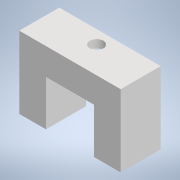
# Autodesk Inventor part: Toper_Carril
Saved by Autodesk Inventor 2022 (Build 260153000, 153)
## iProperties
Created: 2022-01-30
Part Number: Toper_Carril
Material: Generic
Document SubType Name: Modeling
Designer: katha
Density: 1 g/cm^3
Appearance: Default
Author: katha
Autodesk Inventor part; units mm, degrees
ref_plane "YZ Plane" through (0, 0, 0) normal (1, 0, 0) x (0, 1, 0)
ref_plane "XZ Plane" through (0, 0, 0) normal (0, 1, 0) x (-1, 0, 0)
ref_plane "XY Plane" through (0, 0, 0) normal (0, 0, 1) x (1, 0, 0)
sketch "Sketch1" plane through (0, 0, 0) normal (0, 0, 1) x (1, 0, 0)
  line L0 (0, 0) -> (0, 3)
  line L1 (0, 3) -> (25, 3)
  line L2 (25, 3) -> (25, 0)
  line L3 (25, 0) -> (0, 0)
  line L4 (0.5, 3.5) -> (24.5, 3.5)
  line L5 (25, 3) -> (28, 3)
  line L6 (28, 3) -> (28, -17)
  line L7 (28, -17) -> (25, -17)
  line L8 (25, -17) -> (25, 3)
  line L9 (24.5, 3.5) -> (28.5, 3.5)
  line L10 (28.5, 3.5) -> (28.5, -17.5)
  line L11 (28.5, -17.5) -> (24.5, -17.5)
  line L12 (24.5, -17.5) -> (24.5, -0.5)
  line L13 (-3, 3) -> (0, 3)
  line L14 (0, 3) -> (0, -17)
  line L15 (0, -17) -> (-3, -17)
  line L16 (-3, -17) -> (-3, 3)
  line L17 (0.5, 3.5) -> (-3.5, 3.5)
  line L18 (-3.5, 3.5) -> (-3.5, -17.5)
  line L19 (-3.5, -17.5) -> (0.5, -17.5)
  line L20 (24.5, -0.5) -> (0.5, -0.5)
  line L21 (0.5, -17.5) -> (0.5, -0.5)
  line L22 (12.5, 0) -> (12.5, -5.0944) construction
  line L23 (21.5, -3.5) -> (21.5, -20.5)
  line L24 (21.5, -20.5) -> (31.5, -20.5)
  line L25 (31.5, -20.5) -> (31.5, 6.5)
  line L26 (31.5, 6.5) -> (24.5, 6.5)
  line L27 (24.5, 6.5) -> (0.5, 6.5)
  line L28 (0.5, 6.5) -> (-6.5, 6.5)
  line L29 (-6.5, 6.5) -> (-6.5, -20.5)
  line L30 (-6.5, -20.5) -> (3.5, -20.5)
  line L31 (3.5, -20.5) -> (3.5, -3.5)
  line L32 (3.5, -3.5) -> (21.5, -3.5)
  dimension "d1" = 0.5
  dimension "d3" = 0.5
  dimension "d4" = 0.5
  dimension "d5" = 3
  constraints: 66 end point, 8 vertical, 6 horizontal, 3 equal length, 1 midpoint, 22 other
  measures "d1" distance between parallel lines of L8 L12
  measures "d3" distance between parallel lines of L7 L11
  measures "d4" distance between parallel lines of L20 L3
  measures "d5" distance between parallel lines of L12 L23
extrude "Extrusion1" add sketch "Sketch1" against normal blind 10 contours L32 L31 L30 L29 L28 L27 L26 L25 L24 L23
extrude "Extrusion2" add sketch "Sketch1" along normal blind 5 contours L14 L15 L16 L13 L0 | L0 L1 L2 L3 | L2 L5 L6 L7 L8 | L4 L9 L10 L11 L12 L20 L21 L19 L18 L17 | L32 L31 L30 L29 L28 L27 L26 L25 L24 L23
sketch "Sketch2" plane through (3.5, -3.5, -10) normal (0, -1, 0) x (1, 0, 0)
  line L0 (0, 0) -> (-10, 0) projected
  line L1 (18, 15) -> (18, 0) projected
  line L2 (0, 0) -> (18, 0) construction
  line L3 (18, 0) -> (18, 10)
  line L4 (18, 10) -> (0, 10) construction
  line L5 (0, 10) -> (0, 0) construction
  point P0 (-3.5, 10)
  point P1 (9, 5)
  dimension "d10" = 5
  dimension "d11" = 9
  dimension "d12" = 10
  constraints: 8 end point, 2 parallel, 1 horizontal, 1 perpendicular, 1 point on line
  measures "d10" distance from line of L2 point (9, 5)
  measures "d11" distance from line of L5 point (9, 5)
  measures "d12" distance between parallel lines of L4 L2
hole "Hole1" at (12.5, -3.5, -5) direction (0, 1, 0) diameter 5 depth 300 tip angle 118
body "Solid1"
